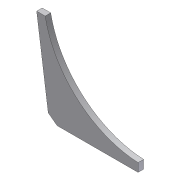
# Autodesk Inventor part: FE-00013-03
Saved by Autodesk Inventor 2012 (Build 160160000, 160)
## iProperties
Created: 2008-05-28
Part Number: FE-00013-03
Document SubType Name: Modeling
Designer: narosenberg
Density: 1 g/cm^3
Description: Gussett
Mass: 24.2355 g
Surface Area: 99.8727 cm^2
Volume: 24.2355 cm^3
Material: Default
Author: narosenberg
Autodesk Inventor part; units mm, degrees
ref_plane "YZ Plane" through (0, 0, 0) normal (1, 0, 0) x (0, 1, 0)
ref_plane "XZ Plane" through (0, 0, 0) normal (0, 1, 0) x (-1, 0, 0)
ref_plane "XY Plane" through (0, 0, 0) normal (0, 0, 1) x (1, 0, 0)
sketch "Sketch1" plane through (0, 0, 0) normal (0, 0, 1) x (1, 0, 0)
  line L0 (-115.1754, 107.4561) -> (0.7036, 107.4561)
  line L1 (0.7036, 107.4561) -> (0.7036, 5.8561)
  line L2 (0.7036, 5.8561) -> (-115.1754, 5.8561)
  line L3 (-115.1754, 5.8561) -> (-115.1754, 107.4561)
  line L4 (-115.1754, 107.4561) -> (-100.8964, 5.8561)
  arc A0 (-105.5234, 107.4561) -> (0.7036, 15.5081) centre (6.6, 129.6559) ccw
  line L5 (-101.9706, 13.4992) -> (-91.8279, 5.8561)
  dimension "d0" = 101.6
  dimension "d2" = 8
  dimension "d6" = 9.652
  dimension "d7" = 9.652
  dimension "d8" = 114.3
  dimension "d9" = 123.7998
  dimension "d13" = 101.6
  dimension "d14" = 12.7
  dimension "d15" = 37
  constraints: 12 end point, 5 point on line, 2 parallel, 2 point on circle, 1 centre point, 1 horizontal, 1 perpendicular
  measures "d0" distance of L0.end L1.end
  measures "d2" angle of L3 L4
  measures "d6" distance of A0.start L0.start
  measures "d7" distance of L1.end A0.end
  measures "d8" radius of A0
  measures "d9" distance from line of L2 A0.centre
  measures "d13" distance of L4.end L1.end
  measures "d14" distance of L5.start L5.end
  measures "d15" angle of L2 L5
extrude "Extrusion1" add sketch "Sketch1" along normal blind 6.35 contours L0 A0 L1 L2 L5 L4
body "Solid1"
